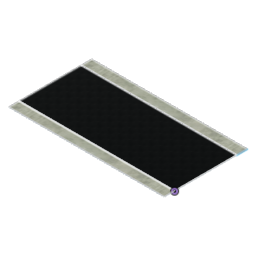
_6ft Extension.78c9b4ef-d159-4e6e-bbc3-9129cdb20226 (Autodesk Fusion 360 design; units mm, degrees)
Autodesk Fusion 360 part; units mm, degrees
sketch "Sketch1" plane through (0, 0, 0) normal (0, 0, 1) x (1, 0, 0)
  line L0 (0, 0) -> (-1524, 0)
  line L1 (-1524, 0) -> (-1524, 609.6)
  line L2 (-1524, 609.6) -> (0, 609.6)
  line L3 (0, 609.6) -> (0, 0)
  line L4 (-1524, 0) -> (0, 0)
  line L5 (0, 0) -> (0, -101.6)
  line L6 (0, -101.6) -> (-1524, -101.6)
  line L7 (-1524, -101.6) -> (-1524, 0)
  line L8 (-1524, 609.6) -> (0, 609.6)
  line L9 (0, 609.6) -> (0, 711.2)
  line L10 (0, 711.2) -> (-1524, 711.2)
  line L11 (-1524, 711.2) -> (-1524, 609.6)
  dimension "d1" = 1524
  dimension "d2" = 609.6
  dimension "d3" = 1524
  dimension "d4" = 101.6
  dimension "d5" = 101.6
  constraint horizontal L0
  constraint vertical L1
  constraint horizontal L2
  constraint vertical L3
  constraint coincident L0.start L3.end
  constraint horizontal L4
  constraint vertical L5
  constraint horizontal L6
  constraint vertical L7
  constraint horizontal L8
  constraint vertical L9
  constraint horizontal L10
  constraint vertical L11
  measures "d1" distance of L0.start L0.end
  measures "d2" distance of L0.start L2.end
  measures "d3" distance of L0.end L0.start
  measures "d4" distance of L0.end L6.end
  measures "d5" distance of L1.end L10.end
extrude "Extrude1" add sketch "Sketch1" along normal blind 6.35 contours L0 L1 L2 L3 L4 L8
extrude "Extrude2" add sketch "Sketch1" along normal blind 6.096 contours L0 L4 L5 L6 L7 | L2 L8 L9 L10 L11
